1.3mm_closer2 (Autodesk Fusion 360 design; units mm, degrees)
Autodesk Fusion 360 part; units mm, degrees
sketch "Sketch1" plane through (0, 0, 0) normal (0, 1, 0) x (1, 0, 0)
  line L0 (0, 0) -> (0, -10)
  line L1 (0, -10) -> (-12.5, -10)
  line L2 (-12.5, -10) -> (-12.5, -7.6)
  line L3 (-12.5, -7.6) -> (-7.5, -7.6)
  line L4 (-7.5, -7.6) -> (-7.5, -0.8)
  line L5 (-7.5, -0.8) -> (-3, -0.8)
  line L6 (-3, -0.8) -> (-3, 0)
  line L7 (-3, 0) -> (0, 0)
  dimension "d1" = 10
  dimension "d2" = 3
  dimension "d4" = 7.6
  dimension "d5" = 5
  dimension "d7" = 0.8
  dimension "d8" = 4.5
  constraint coincident L0.start L7.end
  constraint vertical L0
  constraint perpendicular L0 L1
  constraint perpendicular L1 L2
  constraint perpendicular L0 L3
  constraint perpendicular L1 L4
  constraint perpendicular L4 L5
  constraint perpendicular L1 L6
  constraint perpendicular L0 L7
  measures "d1" distance of L0.start L0.end
  measures "d2" distance of L6.end L0.start
  measures "d4" distance of L0.start L3
  measures "d5" distance of L2.end L3.end
  measures "d7" distance of L0.start L5
  measures "d8" distance of L4.end L5.end
revolve "Revolve1" add sketch "Sketch1" angle 360 about axis through (1.75, 0, 0) along (1, 0, 0)
sketch "Sketch3" plane through (0, 0, 0) normal (1, 0, 0) x (0, 1, 0)
  line L0 (8.0825, 0.0522) -> (-8.0825, -0.0522) construction
  line L1 (-8.0825, -0.0522) -> (-8.0502, -5.0541) construction
  line L2 (-8.0502, -5.0541) -> (8.1148, -4.9497) construction
  line L3 (8.1148, -4.9497) -> (8.0825, 0.0522) construction
  circle A0 centre (0, 0) radius 10
  line L4 (8.0825, 6.3018) -> (-8.0825, 6.1974) construction
  line L5 (-8.0825, 6.1974) -> (-8.0502, 1.1954) construction
  line L6 (-8.0502, 1.1954) -> (8.1148, 1.2998) construction
  line L7 (8.1148, 1.2998) -> (8.0825, 6.3018) construction
  dimension "d13" = 3
  dimension "d20" = 5
  text T0 "1.3 mm" font "Arial" height 3 align centre middle in box 16.1653 x 5.002 at (8.0825, 0.0522) x (-0.999979, -0.006457) y (0.006457, -0.999979) spacing 1
  text T1 "B" font "Arial" height 5 align centre middle in box 16.1653 x 5.002 at (8.0825, 6.3018) x (-0.999979, -0.006457) y (0.006457, -0.999979) spacing 1
  constraint coincident A0.centre
emboss "Emboss1" depth 0.4 profiles "Sketch3" section 1 text T1 T0 onto face at (0, 1.6236, 1.9302)
fillet "Fillet2" radius 0.5 1 edges at (-7.5, -0.2893, -0.7459)
fillet "Fillet1" radius 0.5 3 edges at (-12.5, -3.6162, -9.3233) (-12.5, -2.7483, -7.0857) (0, -3.6162, -9.3233)
equation "d7 = 1.6 mm / 2"
